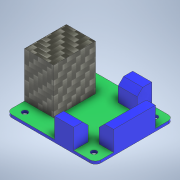
# Autodesk Inventor part: драйвер
Saved by Autodesk Inventor 2022 (Build 260153000, 153)
## iProperties
Created: 2023-05-17
Part Number: драйвер
Material: Типовые
Document SubType Name: Modeling
Designer: korsh624
Density: 1 g/cm^3
Appearance: По умолчанию
Author: korsh624
Autodesk Inventor part; units mm, degrees
ref_plane "YZ Plane" through (0, 0, 0) normal (1, 0, 0) x (0, 1, 0)
ref_plane "XZ Plane" through (0, 0, 0) normal (0, 1, 0) x (-1, 0, 0)
ref_plane "XY Plane" through (0, 0, 0) normal (0, 0, 1) x (1, 0, 0)
sketch "Эскиз1" plane through (0, 0, 0) normal (0, 1, 0) x (-1, 0, 0)
  line L0 (0, 0) -> (49, 0)
  line L1 (49, 0) -> (49, 43)
  line L2 (49, 43) -> (0, 43)
  line L3 (0, 43) -> (0, 0)
  dimension "d0" = 49
  dimension "d1" = 43
  constraints: 8 end point, 2 parallel, 1 horizontal, 1 perpendicular
  measures "d0" distance of L2.end L1.end
  measures "d1" distance of L1.end L0.end
extrude "Выдавливание1" add sketch "Эскиз1" along normal blind 1.5
sketch "Эскиз2" plane through (0, 1.5, 0) normal (0, 1, 0) x (1, 0, 0)
  circle A0 centre (-43.5, -4.7) radius 1.5
  circle A1 centre (-43.5, -38.3) radius 1.5
  circle A2 centre (-5.5, -4.7) radius 1.5
  circle A3 centre (-5.5, -38.3) radius 1.5
  line L0 (-49, 0) -> (-49, -43) projected
  line L1 (0, 0) -> (-49, 0) projected
  line L2 (-49, -43) -> (0, -43) projected
  line L3 (0, -43) -> (0, 0) projected
  dimension "d4" = 3
  dimension "d5" = 3
  dimension "d6" = 3
  dimension "d7" = 3
  dimension "d8" = 5.5
  dimension "d9" = 5.5
  dimension "d10" = 4.7
  dimension "d11" = 4.7
  dimension "d12" = 5.5
  dimension "d13" = 5.5
  dimension "d14" = 4.7
  dimension "d15" = 4.7
  constraints: 4 centre point
  measures "d4" diameter of A0
  measures "d5" diameter of A1
  measures "d6" diameter of A2
  measures "d7" diameter of A3
  measures "d8" distance from line of A0.centre L0
  measures "d9" distance from line of L0 A1.centre
  measures "d10" distance from line of A0.centre L1
  measures "d11" distance from line of A1.centre L2
  measures "d12" distance from line of A2.centre L3
  measures "d13" distance from line of A3.centre L3
  measures "d14" distance from line of L2 A3.centre
  measures "d15" distance from line of A2.centre L1
extrude "Выдавливание2" cut sketch "Эскиз2" against normal blind 1.5 contours A0 | A1 | A2 | A3
sketch "Эскиз3" plane through (0, 1.5, 0) normal (0, 1, 0) x (1, 0, 0)
  line L0 (0, 0) -> (-49, 0) projected
  line L1 (-22.5, 0) -> (-12, 0)
  line L2 (-12, 0) -> (-12, -8)
  line L3 (-12, -8) -> (-22.5, -8)
  line L4 (-22.5, -8) -> (-22.5, 0)
  line L5 (0, -43) -> (0, 0) projected
  line L6 (-49, -43) -> (0, -43) projected
  line L7 (-22.5, -43) -> (-12, -43)
  line L8 (-12, -43) -> (-12, -35)
  line L9 (-12, -35) -> (-22.5, -35)
  line L10 (-22.5, -35) -> (-22.5, -43)
  line L11 (0, -33) -> (-8, -33)
  line L12 (-8, -33) -> (-8, -10)
  line L13 (-8, -10) -> (0, -10)
  line L14 (0, -10) -> (0, -33)
  point P0 (0, -10)
  dimension "d18" = 10.5
  dimension "d19" = 8
  dimension "d20" = 12
  dimension "d21" = 8
  dimension "d22" = 8
  dimension "d23" = 10
  dimension "d24" = 10
  constraints: 24 end point, 6 parallel, 3 horizontal, 3 perpendicular, 3 point on line
  measures "d18" distance of L2.end L3.end
  measures "d19" distance of L3.end L1.start
  measures "d20" distance between parallel lines of L2 L5
  measures "d21" distance between parallel lines of L9 L6
  measures "d22" distance of L12.end L13.end
  measures "d23" distance between parallel lines of L11 L6
  measures "d24" distance between parallel lines of L13 L0
extrude "Выдавливание3" add sketch "Эскиз3" along normal blind 11
chamfer "Фаска1" distance 3 angle 45 3 edges at (-17.25, 12.5, 8) (-17.25, 12.5, 35) (-8, 12.5, 21.5)
fillet "Сопряжение1" radius 3 4 edges at (0, 0.75, 0) (0, 0.75, 43) (-49, 0.75, 43) (-49, 0.75, 0)
sketch "Эскиз4" plane through (0, 1.5, 0) normal (0, 1, 0) x (1, 0, 0)
  line L0 (-49, -3) -> (-49, -40) projected
  line L1 (-49, -33) -> (-33, -33)
  line L2 (-33, -33) -> (-33, -10)
  line L3 (-33, -10) -> (-49, -10)
  line L4 (-49, -10) -> (-49, -33)
  line L5 (-22.5, 0) -> (-46, 0) projected
  line L6 (-46, -43) -> (-22.5, -43) projected
  point P0 (0, 0)
  dimension "d31" = 23
  dimension "d32" = 16
  dimension "d33" = 43
  dimension "d34" = 10
  constraints: 8 end point, 2 parallel, 1 horizontal, 1 perpendicular, 1 point on line
  measures "d31" distance of L1.end L2.end
  measures "d32" distance of L1.start L1.end
  measures "d33" distance between parallel lines of L5 L6
  measures "d34" distance between parallel lines of L6 L1
extrude "Выдавливание4" add sketch "Эскиз4" along normal blind 25
equation "\"d9\" = d8"
equation "\"d11\" = d10"
equation "\"d12\" = d8"
equation "\"d13\" = d12"
equation "\"d14\" = d11"
equation "\"d15\" = d11"
equation "\"d21\" = d19"
